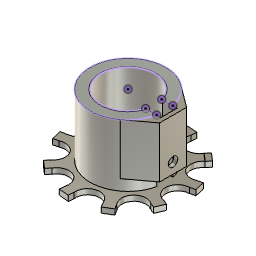
Small gear (Autodesk Fusion 360 design; units mm, degrees)
Autodesk Fusion 360 part; units mm, degrees
sketch "Sketch1" plane through (0, 0, 0) normal (0, 0, 1) x (1, 0, 0)
  circle A0 centre (0, 0) radius 20.2127
  circle A1 centre (7.7908, 18.6509) radius 4.5
  line L0 (11.7242, 16.465) -> (14.5091, 14.0726)
  line L1 (14.5091, 14.0726) -> (15.8123, 15.5897)
  line L2 (11.7242, 16.465) -> (13.0274, 17.9821)
  line L3 (13.0274, 17.9821) -> (15.8123, 15.5897)
  circle A2 centre (-4.6599, 19.6682) radius 4.5
  circle A3 centre (0, 0) radius 20.2127
  circle A4 centre (-15.3306, 13.1729) radius 4.5
  circle A5 centre (0, 0) radius 20.2127
  circle A6 centre (-20.1456, 1.646) radius 4.5
  circle A7 centre (0, 0) radius 20.2127
  circle A8 centre (-17.2656, -10.5096) radius 4.5
  circle A9 centre (0, 0) radius 20.2127
  circle A10 centre (-7.7908, -18.6509) radius 4.5
  circle A11 centre (0, 0) radius 20.2127
  circle A12 centre (4.6599, -19.6682) radius 4.5
  circle A13 centre (0, 0) radius 20.2127
  circle A14 centre (15.3306, -13.1729) radius 4.5
  circle A15 centre (0, 0) radius 20.2127
  circle A16 centre (20.1456, -1.646) radius 4.5
  circle A17 centre (0, 0) radius 20.2127
  circle A18 centre (17.2656, 10.5096) radius 4.5
  circle A19 centre (0, 0) radius 20.2127
  line L4 (-0.1928, 20.2118) -> (-0.0302, 22.2052)
  line L5 (-0.0302, 22.2052) -> (3.629, 21.9066)
  line L6 (3.4664, 19.9132) -> (3.629, 21.9066)
  circle A20 centre (0, 0) radius 20.2127
  line L7 (-12.0362, 16.2383) -> (-13.0763, 17.9466)
  line L8 (-13.0763, 17.9466) -> (-9.9404, 19.8559)
  line L9 (-8.9003, 18.1477) -> (-9.9404, 19.8559)
  circle A21 centre (0, 0) radius 20.2127
  line L10 (-19.2821, 6.0624) -> (-21.1277, 6.8331)
  line L11 (-21.1277, 6.8331) -> (-19.713, 10.2209)
  line L12 (-17.8674, 9.4503) -> (-19.713, 10.2209)
  circle A22 centre (0, 0) radius 20.2127
  line L13 (-19.163, -6.4292) -> (-21.109, -6.8905)
  line L14 (-21.109, -6.8905) -> (-21.9559, -3.3181)
  line L15 (-20.0098, -2.8568) -> (-21.9559, -3.3181)
  circle A23 centre (0, 0) radius 20.2127
  line L16 (-11.7242, -16.465) -> (-13.0274, -17.9821)
  line L17 (-13.0274, -17.9821) -> (-15.8123, -15.5897)
  line L18 (-14.5091, -14.0726) -> (-15.8123, -15.5897)
  circle A24 centre (0, 0) radius 20.2127
  line L19 (0.1928, -20.2118) -> (0.0302, -22.2052)
  line L20 (0.0302, -22.2052) -> (-3.629, -21.9066)
  line L21 (-3.4664, -19.9132) -> (-3.629, -21.9066)
  circle A25 centre (0, 0) radius 20.2127
  line L22 (12.0362, -16.2383) -> (13.0763, -17.9466)
  line L23 (13.0763, -17.9466) -> (9.9404, -19.8559)
  line L24 (8.9003, -18.1477) -> (9.9404, -19.8559)
  circle A26 centre (0, 0) radius 20.2127
  line L25 (19.2821, -6.0624) -> (21.1277, -6.8331)
  line L26 (21.1277, -6.8331) -> (19.713, -10.2209)
  line L27 (17.8674, -9.4503) -> (19.713, -10.2209)
  circle A27 centre (0, 0) radius 20.2127
  line L28 (19.163, 6.4292) -> (21.109, 6.8905)
  line L29 (21.109, 6.8905) -> (21.9559, 3.3181)
  line L30 (20.0098, 2.8568) -> (21.9559, 3.3181)
  circle A28 centre (0, 0) radius 20.2127
  dimension "d1" = 40.4254
  dimension "d2" = 9
  dimension "d11" = 2
  dimension "d12" = 2
  dimension "d14" = 360
  dimension "d16" = 360
  constraint coincident A0.centre A3.centre
  constraint coincident A0 A1.centre
  constraint coincident A1 L0.start
  constraint coincident A0 L0.start
  constraint coincident A0 L0.end
  constraint perpendicular L0 L1
  constraint perpendicular L0 L2
  measures "d1" diameter of A0
  measures "d2" diameter of A1
  measures "d11" distance of L0.end L1.end
  measures "d12" distance of L0.start L2.end
extrude "Extrude1" add sketch "Sketch1" along normal blind 2 contours A0 A1 L0 A2 A3 A4 A5 A6 A7 A8 A9 A10 A11 A12 A13 A14 A15 A16 A17 A18 A19 A20 A21 A22 A23 A24 A25 A26 A27 A28 | A0 A3 A5 A7 A9 A11 A13 A15 A17 A19 A20 A21 A22 A23 A24 A25 A26 A27 L28 L29 L30 A28 | A0 A3 A5 A7 A9 A11 A13 A15 A17 A19 A20 A21 A22 A23 A24 A25 A26 L25 L26 L27 A27 A28 | A0 L1 L2 L3 A3 A5 A7 A9 A11 A13 A15 A17 A19 A20 A21 A22 A23 A24 A25 A26 A27 A28 | A0 A3 A5 A7 A9 A11 A13 A15 A17 A19 A20 A21 A22 A23 A24 A25 L22 L23 L24 A26 A27 A28 | A0 A3 A5 A7 A9 A11 A13 A15 A17 A19 L4 L5 L6 A20 A21 A22 A23 A24 A25 A26 A27 A28 | A0 A3 A5 A7 A9 A11 A13 A15 A17 A19 A20 A21 A22 A23 A24 L19 L20 L21 A25 A26 A27 A28 | A0 A3 A5 A7 A9 A11 A13 A15 A17 A19 A20 L7 L8 L9 A21 A22 A23 A24 A25 A26 A27 A28 | A0 A3 A5 A7 A9 A11 A13 A15 A17 A19 A20 A21 A22 A23 L16 L17 L18 A24 A25 A26 A27 A28 | A0 A3 A5 A7 A9 A11 A13 A15 A17 A19 A20 A21 L10 L11 L12 A22 A23 A24 A25 A26 A27 A28 | A0 A3 A5 A7 A9 A11 A13 A15 A17 A19 A20 A21 A22 L13 L14 L15 A23 A24 A25 A26 A27 A28 makes body 1 at (-1.9939, 0.1629, 0)
sketch "Sketch14" plane through (0, 0, 2) normal (0, 0, 1) x (-1, 0, 0)
  arc A0 (-20.0105, -2.852) -> (-20.0098, -2.8568) centre (0, 0) ccw
  line L0 (-20.0098, -2.8568) -> (-21.9559, -3.3181)
  line L1 (-21.9559, -3.3181) -> (-21.109, -6.8905)
  line L2 (-21.109, -6.8905) -> (-19.163, -6.4292)
  arc A1 (-14.5125, -14.0692) -> (-19.163, -6.4292) centre (-17.2656, -10.5096) ccw
  arc A2 (-14.5125, -14.0692) -> (-14.5091, -14.0726) centre (0, 0) ccw
  line L3 (-14.5091, -14.0726) -> (-11.7242, -16.465)
  arc A3 (-3.4712, -19.9124) -> (-11.7242, -16.465) centre (-7.7908, -18.6509) ccw
  arc A4 (-3.4712, -19.9124) -> (-3.4664, -19.9132) centre (0, 0) ccw
  line L4 (-3.4664, -19.9132) -> (-3.629, -21.9066)
  line L5 (-3.629, -21.9066) -> (0.0302, -22.2052)
  line L6 (0.0302, -22.2052) -> (0.1928, -20.2118)
  arc A5 (8.896, -18.1498) -> (0.1928, -20.2118) centre (4.6599, -19.6682) ccw
  arc A6 (8.896, -18.1498) -> (8.9003, -18.1477) centre (0, 0) ccw
  line L7 (8.9003, -18.1477) -> (9.9404, -19.8559)
  line L8 (9.9404, -19.8559) -> (13.0763, -17.9466)
  line L9 (13.0763, -17.9466) -> (12.0362, -16.2383)
  arc A7 (17.8652, -9.4546) -> (12.0362, -16.2383) centre (15.3306, -13.1729) ccw
  arc A8 (17.8652, -9.4546) -> (17.8674, -9.4503) centre (0, 0) ccw
  line L10 (17.8674, -9.4503) -> (19.713, -10.2209)
  line L11 (19.713, -10.2209) -> (21.1277, -6.8331)
  line L12 (21.1277, -6.8331) -> (19.2821, -6.0624)
  arc A9 (20.0105, 2.852) -> (19.2821, -6.0624) centre (20.1456, -1.646) ccw
  arc A10 (20.0105, 2.852) -> (20.0098, 2.8568) centre (0, 0) ccw
  line L13 (20.0098, 2.8568) -> (21.9559, 3.3181)
  line L14 (21.9559, 3.3181) -> (21.109, 6.8905)
  line L15 (21.109, 6.8905) -> (19.163, 6.4292)
  arc A11 (14.5125, 14.0692) -> (19.163, 6.4292) centre (17.2656, 10.5096) ccw
  arc A12 (14.5125, 14.0692) -> (14.5091, 14.0726) centre (0, 0) ccw
  line L16 (14.5091, 14.0726) -> (15.8123, 15.5897)
  line L17 (15.8123, 15.5897) -> (13.0274, 17.9821)
  line L18 (13.0274, 17.9821) -> (11.7242, 16.465)
  arc A13 (3.4712, 19.9124) -> (11.7242, 16.465) centre (7.7908, 18.6509) ccw
  arc A14 (3.4712, 19.9124) -> (3.4664, 19.9132) centre (0, 0) ccw
  line L19 (3.4664, 19.9132) -> (3.629, 21.9066)
  line L20 (3.629, 21.9066) -> (-0.0302, 22.2052)
  line L21 (-0.0302, 22.2052) -> (-0.1928, 20.2118)
  arc A15 (-8.896, 18.1498) -> (-0.1928, 20.2118) centre (-4.6599, 19.6682) ccw
  arc A16 (-8.896, 18.1498) -> (-8.9003, 18.1477) centre (0, 0) ccw
  line L22 (-8.9003, 18.1477) -> (-9.9404, 19.8559)
  line L23 (-9.9404, 19.8559) -> (-13.0763, 17.9466)
  line L24 (-13.0763, 17.9466) -> (-12.0362, 16.2383)
  arc A17 (-17.8652, 9.4546) -> (-12.0362, 16.2383) centre (-15.3306, 13.1729) ccw
  arc A18 (-17.8652, 9.4546) -> (-17.8674, 9.4503) centre (0, 0) ccw
  line L25 (-17.8674, 9.4503) -> (-19.713, 10.2209)
  line L26 (-19.713, 10.2209) -> (-21.1277, 6.8331)
  line L27 (-21.1277, 6.8331) -> (-19.2821, 6.0624)
  arc A19 (-20.0105, -2.852) -> (-19.2821, 6.0624) centre (-20.1456, 1.646) ccw
  circle A20 centre (-7, 0) radius 2
  circle A21 centre (7, 0) radius 2
  dimension "d57" = 4
  measures "d57" diameter of A20
extrude "Extrude12" cut sketch "Sketch14" against normal blind 3 contours A20 | A21 bodies 1
sketch "Sketch4" plane through (0, 0, 2) normal (0, 0, 1) x (-1, 0, 0)
  arc A0 (-20.0105, -2.852) -> (-20.0098, -2.8568) centre (0, 0) ccw
  line L0 (-20.0098, -2.8568) -> (-21.9559, -3.3181)
  line L1 (-21.9559, -3.3181) -> (-21.109, -6.8905)
  line L2 (-21.109, -6.8905) -> (-19.163, -6.4292)
  arc A1 (-14.5125, -14.0692) -> (-19.163, -6.4292) centre (-17.2656, -10.5096) ccw
  arc A2 (-14.5125, -14.0692) -> (-14.5091, -14.0726) centre (0, 0) ccw
  line L3 (-14.5091, -14.0726) -> (-11.7242, -16.465)
  arc A3 (-3.4712, -19.9124) -> (-11.7242, -16.465) centre (-7.7908, -18.6509) ccw
  arc A4 (-3.4712, -19.9124) -> (-3.4664, -19.9132) centre (0, 0) ccw
  line L4 (-3.4664, -19.9132) -> (-3.629, -21.9066)
  line L5 (-3.629, -21.9066) -> (0.0302, -22.2052)
  line L6 (0.0302, -22.2052) -> (0.1928, -20.2118)
  arc A5 (8.896, -18.1498) -> (0.1928, -20.2118) centre (4.6599, -19.6682) ccw
  arc A6 (8.896, -18.1498) -> (8.9003, -18.1477) centre (0, 0) ccw
  line L7 (8.9003, -18.1477) -> (9.9404, -19.8559)
  line L8 (9.9404, -19.8559) -> (13.0763, -17.9466)
  line L9 (13.0763, -17.9466) -> (12.0362, -16.2383)
  arc A7 (17.8652, -9.4546) -> (12.0362, -16.2383) centre (15.3306, -13.1729) ccw
  arc A8 (17.8652, -9.4546) -> (17.8674, -9.4503) centre (0, 0) ccw
  line L10 (17.8674, -9.4503) -> (19.713, -10.2209)
  line L11 (19.713, -10.2209) -> (21.1277, -6.8331)
  line L12 (21.1277, -6.8331) -> (19.2821, -6.0624)
  arc A9 (20.0105, 2.852) -> (19.2821, -6.0624) centre (20.1456, -1.646) ccw
  arc A10 (20.0105, 2.852) -> (20.0098, 2.8568) centre (0, 0) ccw
  line L13 (20.0098, 2.8568) -> (21.9559, 3.3181)
  line L14 (21.9559, 3.3181) -> (21.109, 6.8905)
  line L15 (21.109, 6.8905) -> (19.163, 6.4292)
  arc A11 (14.5125, 14.0692) -> (19.163, 6.4292) centre (17.2656, 10.5096) ccw
  arc A12 (14.5125, 14.0692) -> (14.5091, 14.0726) centre (0, 0) ccw
  line L16 (14.5091, 14.0726) -> (15.8123, 15.5897)
  line L17 (15.8123, 15.5897) -> (13.0274, 17.9821)
  line L18 (13.0274, 17.9821) -> (11.7242, 16.465)
  arc A13 (3.4712, 19.9124) -> (11.7242, 16.465) centre (7.7908, 18.6509) ccw
  arc A14 (3.4712, 19.9124) -> (3.4664, 19.9132) centre (0, 0) ccw
  line L19 (3.4664, 19.9132) -> (3.629, 21.9066)
  line L20 (3.629, 21.9066) -> (-0.0302, 22.2052)
  line L21 (-0.0302, 22.2052) -> (-0.1928, 20.2118)
  arc A15 (-8.896, 18.1498) -> (-0.1928, 20.2118) centre (-4.6599, 19.6682) ccw
  arc A16 (-8.896, 18.1498) -> (-8.9003, 18.1477) centre (0, 0) ccw
  line L22 (-8.9003, 18.1477) -> (-9.9404, 19.8559)
  line L23 (-9.9404, 19.8559) -> (-13.0763, 17.9466)
  line L24 (-13.0763, 17.9466) -> (-12.0362, 16.2383)
  arc A17 (-17.8652, 9.4546) -> (-12.0362, 16.2383) centre (-15.3306, 13.1729) ccw
  arc A18 (-17.8652, 9.4546) -> (-17.8674, 9.4503) centre (0, 0) ccw
  line L25 (-17.8674, 9.4503) -> (-19.713, 10.2209)
  line L26 (-19.713, 10.2209) -> (-21.1277, 6.8331)
  line L27 (-21.1277, 6.8331) -> (-19.2821, 6.0624)
  arc A19 (-20.0105, -2.852) -> (-19.2821, 6.0624) centre (-20.1456, 1.646) ccw
  circle A20 centre (0, 0) radius 10
  circle A21 centre (7, 0) radius 2
  circle A22 centre (-7, 0) radius 2
  dimension "d23" = 20
  constraint coincident A0.centre A2.centre
  measures "d23" diameter of A20
sketch "Sketch5" plane through (0, 0, 2) normal (0, 0, 1) x (-1, 0, 0)
extrude "Extrude4" cut sketch "Sketch4" against normal blind 2 contours A20 | A21 | A22 bodies 1
sketch "Sketch8" plane through (0, 0, 2) normal (0, 0, 1) x (-1, 0, 0)
  circle A0 centre (0, 0) radius 10
  arc A1 (-20.0105, -2.852) -> (-20.0098, -2.8568) centre (0, 0) ccw
  line L0 (-20.0098, -2.8568) -> (-21.9559, -3.3181)
  line L1 (-21.9559, -3.3181) -> (-21.109, -6.8905)
  line L2 (-21.109, -6.8905) -> (-19.163, -6.4292)
  arc A2 (-14.5125, -14.0692) -> (-19.163, -6.4292) centre (-17.2656, -10.5096) ccw
  arc A3 (-14.5125, -14.0692) -> (-14.5091, -14.0726) centre (0, 0) ccw
  line L3 (-14.5091, -14.0726) -> (-11.7242, -16.465)
  arc A4 (-3.4712, -19.9124) -> (-11.7242, -16.465) centre (-7.7908, -18.6509) ccw
  arc A5 (-3.4712, -19.9124) -> (-3.4664, -19.9132) centre (0, 0) ccw
  line L4 (-3.4664, -19.9132) -> (-3.629, -21.9066)
  line L5 (-3.629, -21.9066) -> (0.0302, -22.2052)
  line L6 (0.0302, -22.2052) -> (0.1928, -20.2118)
  arc A6 (8.896, -18.1498) -> (0.1928, -20.2118) centre (4.6599, -19.6682) ccw
  arc A7 (8.896, -18.1498) -> (8.9003, -18.1477) centre (0, 0) ccw
  line L7 (8.9003, -18.1477) -> (9.9404, -19.8559)
  line L8 (9.9404, -19.8559) -> (13.0763, -17.9466)
  line L9 (13.0763, -17.9466) -> (12.0362, -16.2383)
  arc A8 (17.8652, -9.4546) -> (12.0362, -16.2383) centre (15.3306, -13.1729) ccw
  arc A9 (17.8652, -9.4546) -> (17.8674, -9.4503) centre (0, 0) ccw
  line L10 (17.8674, -9.4503) -> (19.713, -10.2209)
  line L11 (19.713, -10.2209) -> (21.1277, -6.8331)
  line L12 (21.1277, -6.8331) -> (19.2821, -6.0624)
  arc A10 (20.0105, 2.852) -> (19.2821, -6.0624) centre (20.1456, -1.646) ccw
  arc A11 (20.0105, 2.852) -> (20.0098, 2.8568) centre (0, 0) ccw
  line L13 (20.0098, 2.8568) -> (21.9559, 3.3181)
  line L14 (21.9559, 3.3181) -> (21.109, 6.8905)
  line L15 (21.109, 6.8905) -> (19.163, 6.4292)
  arc A12 (14.5125, 14.0692) -> (19.163, 6.4292) centre (17.2656, 10.5096) ccw
  arc A13 (14.5125, 14.0692) -> (14.5091, 14.0726) centre (0, 0) ccw
  line L16 (14.5091, 14.0726) -> (15.8123, 15.5897)
  line L17 (15.8123, 15.5897) -> (13.0274, 17.9821)
  line L18 (13.0274, 17.9821) -> (11.7242, 16.465)
  arc A14 (3.4712, 19.9124) -> (11.7242, 16.465) centre (7.7908, 18.6509) ccw
  arc A15 (3.4712, 19.9124) -> (3.4664, 19.9132) centre (0, 0) ccw
  line L19 (3.4664, 19.9132) -> (3.629, 21.9066)
  line L20 (3.629, 21.9066) -> (-0.0302, 22.2052)
  line L21 (-0.0302, 22.2052) -> (-0.1928, 20.2118)
  arc A16 (-8.896, 18.1498) -> (-0.1928, 20.2118) centre (-4.6599, 19.6682) ccw
  arc A17 (-8.896, 18.1498) -> (-8.9003, 18.1477) centre (0, 0) ccw
  line L22 (-8.9003, 18.1477) -> (-9.9404, 19.8559)
  line L23 (-9.9404, 19.8559) -> (-13.0763, 17.9466)
  line L24 (-13.0763, 17.9466) -> (-12.0362, 16.2383)
  arc A18 (-17.8652, 9.4546) -> (-12.0362, 16.2383) centre (-15.3306, 13.1729) ccw
  arc A19 (-17.8652, 9.4546) -> (-17.8674, 9.4503) centre (0, 0) ccw
  line L25 (-17.8674, 9.4503) -> (-19.713, 10.2209)
  line L26 (-19.713, 10.2209) -> (-21.1277, 6.8331)
  line L27 (-21.1277, 6.8331) -> (-19.2821, 6.0624)
  arc A20 (-20.0105, -2.852) -> (-19.2821, 6.0624) centre (-20.1456, 1.646) ccw
  circle A21 centre (0, 0) radius 14
  constraint concentric A0 A21
extrude "Extrude7" add sketch "Sketch8" along normal blind 23 separate body contours A21 makes body 2
sketch "Sketch9" plane through (0, 0, 0) normal (1, 0, 0) x (0, 1, 0)
  line L0 (0, 1.8522) -> (0, 25.8522)
  line L1 (-3, 25.7045) -> (3, 25.7045)
  line L2 (3, 25.7045) -> (3, 2)
  line L3 (3, 2) -> (-3, 2)
  line L4 (-3, 2) -> (-3, 25.7045)
  line L5 (-3, 25.7045) -> (3, 2) construction
  line L6 (3, 25.7045) -> (-3, 2) construction
  point P0 (0, 13.8522)
  dimension "d35" = 24
  dimension "d36" = 6
  constraint vertical L0
  constraint horizontal L1
  constraint perpendicular L1 L2
  constraint parallel L1 L3
  constraint parallel L2 L4
  constraint coincident L5 P0
  constraint coincident L6 P0
  constraint midpoint L0 P0
  measures "d35" distance of L0.start L0.end
  measures "d36" distance of L2.end L3.end
extrude "Extrude8" cut sketch "Sketch9" along normal blind 20 bodies 2
sketch "Sketch10" plane through (0, 0, 25) normal (0, 0, 1) x (-1, 0, 0)
  line L0 (-13.6748, 3) -> (-9.5394, 3)
  arc A0 (-9.5394, -3) -> (-9.5394, 3) centre (0, 0) ccw
  line L1 (-9.5394, -3) -> (-13.6748, -3)
  arc A1 (-13.6748, -3) -> (-13.6748, 3) centre (0, 0) ccw
sketch "Sketch11" plane through (0, 0, 25) normal (0, 0, 1) x (-1, 0, 0)
  circle A0 centre (0, 0) radius 10
  circle A1 centre (0, 0) radius 14
  line L0 (-9.5452, 2.9816) -> (-15.2452, 2.9816)
  line L1 (-9.5283, -3.0351) -> (-15.2283, -3.0351)
  line L2 (-15.2283, -3.0351) -> (-15.2452, 2.9816)
  line L3 (-9.5283, -3.0351) -> (-9.5283, -5.0351)
  line L4 (-9.5283, -5.0351) -> (-13.0632, -5.0351)
  line L5 (-16.7283, -4.358) -> (-16.7283, -5.0351)
  line L6 (-16.7283, -5.0351) -> (-13.0632, -5.0351)
  line L7 (-9.5452, 2.9816) -> (-9.5452, 4.9816)
  line L8 (-9.5452, 4.9816) -> (-13.0837, 4.9816)
  line L9 (-13.0837, 4.9816) -> (-16.7283, 4.9816)
  line L10 (-16.7283, 4.9816) -> (-16.7283, -4.358)
  line L11 (-16.7283, 4.9816) -> (-8.3761, 11.2179)
  line L12 (-16.7283, -5.0351) -> (-8.3298, -11.2523)
  dimension "d39" = 28
  dimension "d41" = 5.7
  dimension "d42" = 5.7
  dimension "d43" = 2
  dimension "d45" = 2
  dimension "d56" = 1.5
  constraint coincident A0.centre A1.centre
  constraint concentric A0 A1
  constraint coincident A0 L0.start
  constraint horizontal L0
  constraint coincident A0 L1.start
  constraint horizontal L1
  constraint perpendicular L1 L3
  constraint coincident A1 L4.end
  constraint perpendicular L3 L4
  constraint perpendicular L4 L5
  constraint perpendicular L5 L6
  constraint perpendicular L0 L7
  constraint coincident A1 L8.end
  constraint perpendicular L5 L8
  constraint perpendicular L5 L9
  constraint parallel L5 L10
  constraint coincident A1 L11.end
  constraint tangent A1 L11
  constraint coincident A1 L12.end
  constraint tangent A1 L12
  measures "d39" diameter of A1
  measures "d41" distance of L0.start L0.end
  measures "d42" distance of L1.start L1.end
  measures "d43" distance of L1.start L3.end
  measures "d45" distance of L0.start L7.end
  measures "d56" horizontal distance of L1.end L5.start
extrude "Extrude9" add sketch "Sketch11" against normal blind 19 contours A1 L0 L1 L2 L5 L6 L9 L10 | A1 L9 L11 | A1 L6 L12 bodies 2
sketch "Sketch12" plane through (16.7283, 0, 0) normal (1, 0, 0) x (0, 1, 0)
  line L0 (5.0351, 25) -> (-4.9816, 25)
  line L1 (-4.9816, 6) -> (5.0351, 6)
  circle A0 centre (0, 10) radius 1.75
  line L2 (14, 2) -> (-14, 2)
  line L3 (-4.9816, 25) -> (-4.9816, 6)
  line L4 (5.0351, 6) -> (5.0351, 25)
  dimension "d48" = 3.5
  dimension "d49" = 8
  measures "d48" diameter of A0
  measures "d49" distance of A0.centre L2
extrude "Extrude10" cut sketch "Sketch12" against normal blind 3 contours A0 bodies 2
sketch "Sketch13" plane through (0, 0, 25) normal (0, 0, 1) x (-1, 0, 0)
  circle A0 centre (0, 0) radius 10.25
  dimension "d52" = 20.5
  constraint coincident A0.centre origin
  measures "d52" diameter of A0
extrude "Extrude11" cut sketch "Sketch13" against normal blind 30 bodies 1 2
equation "d41 = 5.2 mm + 0.5 mm"
equation "d46 = -23 mm + 4 mm"
